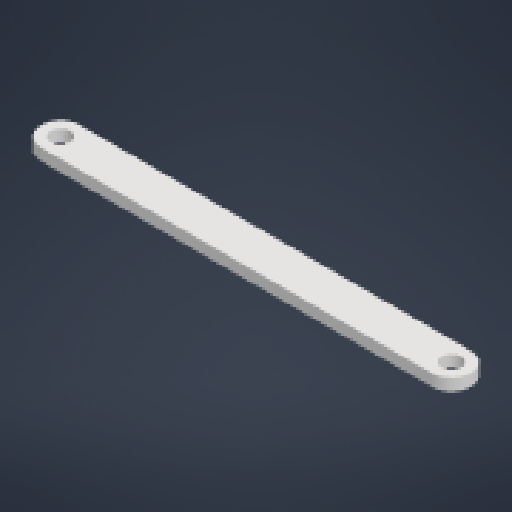
# Autodesk Inventor part: Claw Arm
Saved by Autodesk Inventor 2023.6 (Build 276521000, 521)
## iProperties
Created: 2026-03-05
Part Number: Claw Arm
Material: Generic
Document SubType Name: Modeling
Designer: user
Density: 1 g/cm^3
Appearance: Default
Author: user
Autodesk Inventor part; units mm, degrees
ref_plane "YZ Plane" through (0, 0, 0) normal (1, 0, 0) x (0, 1, 0)
ref_plane "XZ Plane" through (0, 0, 0) normal (0, 1, 0) x (-1, 0, 0)
ref_plane "XY Plane" through (0, 0, 0) normal (0, 0, 1) x (1, 0, 0)
sketch "Sketch1" plane through (0, 0, 0) normal (0, 1, 0) x (-1, 0, 0)
  line L0 (40, 0) -> (-40, 0) construction
  line L1 (40, 5) -> (-40, 5)
  line L2 (-40, -5) -> (40, -5)
  arc A0 (40, -5) -> (40, 5) centre (40, 0) ccw
  arc A1 (-40, 5) -> (-40, -5) centre (-40, 0) ccw
  circle A2 centre (40, 0) radius 2.5
  circle A3 centre (-40, 0) radius 2.5
  point P0 (0, 0)
  dimension "d0" = 40
  dimension "d2" = 5
  dimension "d3" = 5
  constraints: 8 end point, 4 centre point, 4 point on circle, 4 tangent, 2 coincident, 1 horizontal, 1 midpoint, 1 parallel
  measures "d0" distance of point (0, 0) L0.end
  measures "d2" diameter of A2
  measures "d3" diameter of A3
extrude "Extrusion1" add sketch "Sketch1" along normal blind 3
body "Solid1"
